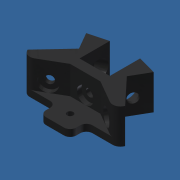
# Autodesk Inventor part: hexagon_top_v_2_0_x1
Saved by Autodesk Inventor 2014 SP2 (Build 180246200, 246)
## iProperties
Created: 2013-09-01
Part Number: hexagon_top_v_2_0_x1
Material: ABS-Kunststoff - Schwarz
Document SubType Name: Modeling
Designer: gerdkeller
Density: 1.06 g/cm^3
Appearance: Glatt - weiß(2)
Author: gerdkeller
Autodesk Inventor part; units mm, degrees
sketch "Skizze1" plane through (0, 0, 0) normal (0, 0, 1) x (1, 0, 0)
  line L0 (10, 10) -> (10, -10)
  line L1 (10, -10) -> (-10, -10)
  line L2 (-10, -10) -> (-10, 10)
  line L3 (0, 8) -> (17.3205, -2) construction
  line L4 (0, 8) -> (20, 8) construction
  line L5 (17.3205, -2) -> (12.3205, -10.6603) construction
  line L6 (17.3205, -2) -> (22.3205, 6.6603) construction
  line L7 (22.3205, 6.6603) -> (12.3205, -10.6603)
  line L8 (12.3205, -10.6603) -> (32.2391, -22.1603)
  line L9 (10, -10) -> (10, -20) construction
  line L10 (-10, -10) -> (-10, -20) construction
  line L11 (29.2391, -27.3564) -> (10, -16.2487)
  line L12 (10, -16.2487) -> (-10, -16.2487)
  line L13 (29.2391, -27.3564) -> (32.2391, -22.1603)
  line L14 (10, 10) -> (22.3205, 6.6603)
  line L15 (0, 17.4713) -> (0, -34.8277) projected
  line L16 (-45.1347, 0) -> (45.1347, 0) projected
  line L17 (-17.3205, -2) -> (-12.3205, -10.6603) construction
  line L18 (-17.3205, -2) -> (-22.3205, 6.6603) construction
  line L19 (-22.3205, 6.6603) -> (-12.3205, -10.6603)
  line L20 (-12.3205, -10.6603) -> (-32.2391, -22.1603)
  line L21 (-29.2391, -27.3564) -> (-10, -16.2487)
  line L22 (-29.2391, -27.3564) -> (-32.2391, -22.1603)
  line L23 (-10, 10) -> (-22.3205, 6.6603)
  point P0 (0, 0)
  dimension "d0" = 20
  dimension "d2" = 20
  dimension "d3" = 30
  dimension "d4" = 10
  dimension "d5" = 10
  dimension "d6" = 23
  dimension "d7" = 6
  dimension "d28" = 10
  dimension "d29" = 8
  dimension "d30" = 16.2487
  dimension "d31" = 30
  dimension "d32" = 14.833
  dimension "d101" = 17.3205
  constraints: 44 end point, 5 symmetric about line, 3 parallel, 3 perpendicular, 2 collinear, 2 point on line, 1 equal length, 1 horizontal, 2 other
  measures "d0" distance between parallel lines of L0 L2
  measures "d2" distance of L3.start L3.end
  measures "d3" angle of L3 L4
  measures "d4" distance of L3.end L5.end
  measures "d5" distance of L3.end L6.end
  measures "d6" distance of L5.end L8.end
  measures "d7" distance between parallel lines of L8 L11
  measures "d28" distance between parallel lines of L1 L16
  measures "d29" distance from line of L16 L3.start
  measures "d30" distance between parallel lines of L12 L16
  measures "d31" angle of L16 L8
  measures "d32" angle of L3 L14
  measures "d101" distance from line of L3.end L15
extrude "Extrusion1" add sketch "Skizze1" along normal blind 40 contours L14 L7 L16 L0 | L16 L7 L8 L13 L11 L12 L15 L1 L0 | L15 L12 L21 L22 L20 L19 L16 L2 L1 | L16 L19 L23 L2
sketch "Skizze5" plane through (0, 0, 0) normal (0, 0, -1) x (-1, 0, 0)
  line L0 (10, 10) -> (10, -10) projected
  line L1 (10, -10) -> (-10, -10) projected
  line L2 (-10, -10) -> (-10, 10) projected
  line L3 (-10, 10) -> (-22.3205, 6.6603) projected
  line L4 (-22.3205, 6.6603) -> (-12.3205, -10.6603) projected
  line L5 (-12.3205, -10.6603) -> (-32.2391, -22.1603) projected
  line L6 (-32.2391, -22.1603) -> (-29.2391, -27.3564) projected
  line L7 (-29.2391, -27.3564) -> (-10, -16.2487) projected
  line L8 (-10, -16.2487) -> (10, -16.2487) projected
  line L9 (10, -16.2487) -> (29.2391, -27.3564) projected
  line L10 (29.2391, -27.3564) -> (32.2391, -22.1603) projected
  line L11 (32.2391, -22.1603) -> (12.3205, -10.6603) projected
  line L12 (12.3205, -10.6603) -> (22.3205, 6.6603) projected
  line L13 (22.3205, 6.6603) -> (10, 10) projected
  line L14 (-10, 10) -> (10, 10)
  line L15 (32.2391, -22.1603) -> (42.2391, -4.8397)
  line L16 (42.2391, -4.8397) -> (22.3205, 6.6603)
  line L17 (-32.2391, -22.1603) -> (-42.2391, -4.8397)
  line L18 (-42.2391, -4.8397) -> (-22.3205, 6.6603)
  point P0 (0, 0)
  dimension "d33" = 20
  dimension "d34" = 20
  constraints: 10 end point, 2 parallel, 1 perpendicular
  measures "d33" distance of L10.end L15.end
  measures "d34" distance of L5.end L17.end
extrude "Extrusion5" add sketch "Skizze5" along normal blind 6
sketch "Skizze6" plane through (0, 0, 0) normal (0, 0, 1) x (1, 0, 0)
  line L0 (42.2391, -4.8397) -> (32.2391, -22.1603) projected
  line L1 (22.3205, 6.6603) -> (42.2391, -4.8397) projected
  circle A0 centre (27.2798, -7.75) radius 2.6
  point P0 (0, 0)
  dimension "d37" = 5.2
  dimension "d38" = 10
  dimension "d39" = 11.5
  constraints: 1 centre point
  measures "d37" diameter of A0
  measures "d38" distance from line of A0.centre L1
  measures "d39" distance from line of L0 A0.centre
extrude "Extrusion6" cut sketch "Skizze6" against normal blind 6
sketch "Skizze7" plane through (0, 0, -6) normal (0, 0, -1) x (-1, 0, 0)
  circle A0 centre (-27.2798, -7.75) radius 2.6 projected
  circle A1 centre (-27.2798, -7.75) radius 5.5
  point P0 (0, 0)
  dimension "d42" = 11
  constraints: 1 centre point, 1 coincident
  measures "d42" diameter of A1
extrude "Extrusion7" cut sketch "Skizze7" against normal blind 3
sketch "Skizze8" plane through (27.2798, -7.75, -3) normal (0, 0, -1) x (-1, 0, 0)
  circle A0 centre (0, 0) radius 2.6 projected
  point P0 (27.2798, 7.75)
extrude "Extrusion8" add sketch "Skizze8" against normal blind 0.4
mirror "Spiegeln1" about plane through (0, 0, 0) normal (1, 0, 0) of "Extrusion6", "Extrusion7", "Extrusion8"
sketch "Skizze9" plane through (12.3205, -10.6603, 40) normal (0.5, 0.8660254, 0) x (0.8660254, -0.5, 0)
  circle A0 centre (11.5, 10) radius 2.6
  point P0 (-16, 40)
  dimension "d47" = 5.2
  constraints: 1 centre point
  measures "d47" diameter of A0
extrude "Extrusion9" cut sketch "Skizze9" against normal blind 6
sketch "Skizze10" plane through (29.2391, -27.3564, -6) normal (-0.5, -0.8660254, 0) x (0.8660254, -0.5, 0)
  circle A0 centre (-11.5, 36) radius 2.6 projected
  circle A1 centre (-11.5, 36) radius 5.5
  point P0 (-39, 6)
  dimension "d50" = 11
  constraints: 1 centre point, 1 coincident
  measures "d50" diameter of A1
extrude "Extrusion10" cut sketch "Skizze10" against normal blind 3
mirror "Spiegeln2" about plane through (0, 0, 0) normal (1, 0, 0) of "Extrusion10", "Extrusion9"
sketch "Skizze12" plane through (0, 0, -6) normal (0, 0, -1) x (-1, 0, 0)
  line L0 (-10, -16.2487) -> (10, -16.2487) projected
  line L1 (10, 10) -> (-10, 10) projected
  line L2 (-10, -16.2487) -> (-10, -36.2487)
  line L3 (-10, -36.2487) -> (10, -36.2487)
  line L4 (10, -36.2487) -> (10, -16.2487)
  point P0 (0, 0)
  dimension "d55" = 20
  constraints: 6 end point, 3 perpendicular
  measures "d55" distance of L0.start L2.end
extrude "Extrusion12" add sketch "Skizze12" against normal blind 6
sketch "Skizze13" plane through (0, 0, 0) normal (0, 0, 1) x (1, 0, 0)
  line L0 (-10, -36.2487) -> (10, -36.2487) projected
  circle A0 centre (0, -26.2487) radius 2.6
  point P0 (0, 0)
  dimension "d58" = 5.2
  dimension "d59" = 10
  constraints: 1 centre point
  measures "d58" diameter of A0
  measures "d59" distance from line of L0 A0.centre
extrude "Extrusion13" cut sketch "Skizze13" against normal blind 6
sketch "Skizze14" plane through (0, 0, -6) normal (0, 0, -1) x (-1, 0, 0)
  circle A0 centre (0, -26.2487) radius 2.6 projected
  circle A1 centre (0, -26.2487) radius 5.5
  point P0 (0, 0)
  dimension "d62" = 11
  constraints: 1 centre point, 1 coincident
  measures "d62" diameter of A1
extrude "Extrusion14" cut sketch "Skizze14" against normal blind 3
sketch "Skizze15" plane through (0, -26.2487, -3) normal (0, 0, -1) x (-1, 0, 0)
  circle A0 centre (0, 0) radius 2.6 projected
  point P0 (0, 26.2487)
extrude "Extrusion15" add sketch "Skizze15" against normal blind 0.4
fillet "Rundung1" radius 5 2 edges at (10, -16.2487, -3) (-10, -16.2487, -3)
sketch "Skizze16" plane through (0, 0, 0) normal (0, 0, 1) x (1, 0, 0)
  circle A0 centre (0, 0) radius 2.6
  dimension "d68" = 5.2
  constraints: 1 centre point, 1 coincident
  measures "d68" diameter of A0
extrude "Extrusion16" cut sketch "Skizze16" against normal blind 6
sketch "Skizze17" plane through (0, 0, -6) normal (0, 0, -1) x (-1, 0, 0)
  circle A0 centre (0, 0) radius 2.6 projected
  circle A1 centre (0, 0) radius 5.5
  dimension "d71" = 11
  constraints: 1 centre point, 1 coincident
  measures "d71" diameter of A1
extrude "Extrusion17" cut sketch "Skizze17" against normal blind 3
sketch "Skizze18" plane through (0, 0, -3) normal (0, 0, -1) x (-1, 0, 0)
  circle A0 centre (0, 0) radius 2.6 projected
extrude "Extrusion18" add sketch "Skizze18" against normal blind 0.4
sketch "Skizze19" plane through (-10, -16.2487, 40) normal (0, -1, 0) x (1, 0, 0)
  circle A0 centre (10, -10) radius 2.6
  point P0 (10, -40)
  dimension "d76" = 5.2
  constraints: 1 centre point
  measures "d76" diameter of A0
extrude "Extrusion19" cut sketch "Skizze19" against normal blind 7
sketch "Skizze20" plane through (-10, -16.2487, 40) normal (0, -1, 0) x (1, 0, 0)
  circle A0 centre (10, -10) radius 2.6 projected
  circle A1 centre (10, -10) radius 5.5
  point P0 (10, -40)
  dimension "d79" = 11
  constraints: 1 centre point, 1 coincident
  measures "d79" diameter of A1
extrude "Extrusion20" cut sketch "Skizze20" against normal blind 3
sketch "Skizze21" plane through (-10, -16.2487, 40) normal (0, -1, 0) x (1, 0, 0)
  circle A0 centre (10, -10) radius 5.5 projected
  circle A1 centre (10, -30) radius 2.6
  point P0 (10, -40)
  dimension "d82" = 5.2
  dimension "d83" = 20
  constraints: 1 centre point
  measures "d82" diameter of A1
  measures "d83" distance of A1.centre A0.centre
extrude "Extrusion21" cut sketch "Skizze21" against normal blind 10 contours A1
sketch "Skizze22" plane through (-10, -16.2487, 40) normal (0, -1, 0) x (1, 0, 0)
  circle A0 centre (10, -30) radius 2.6 projected
  circle A1 centre (10, -30) radius 5.5
  point P0 (10, -40)
  dimension "d86" = 11
  constraints: 1 centre point, 1 coincident
  measures "d86" diameter of A1
extrude "Extrusion22" cut sketch "Skizze22" against normal blind 3
sketch "Skizze23" plane through (29.2391, -27.3564, -6) normal (-0.5, -0.8660254, 0) x (0.8660254, -0.5, 0)
  line L0 (0, 46) -> (0, 0) projected
  circle A0 centre (-11.5, 36) radius 5.5 projected
  circle A1 centre (-11.5, 16) radius 2.6
  point P0 (-39, 6)
  dimension "d89" = 5.2
  dimension "d90" = 20
  dimension "d91" = 11.5
  constraints: 1 centre point
  measures "d89" diameter of A1
  measures "d90" distance of A1.centre A0.centre
  measures "d91" distance from line of L0 A1.centre
extrude "Extrusion23" cut sketch "Skizze23" against normal blind 10 contours A1
sketch "Skizze24" plane through (29.2391, -27.3564, -6) normal (-0.5, -0.8660254, 0) x (0.8660254, -0.5, 0)
  circle A0 centre (-11.5, 16) radius 2.6 projected
  circle A1 centre (-11.5, 16) radius 5.5
  point P0 (-39, 6)
  dimension "d94" = 11
  constraints: 1 centre point, 1 coincident
  measures "d94" diameter of A1
extrude "Extrusion24" cut sketch "Skizze24" against normal blind 3
mirror "Spiegeln3" about plane through (0, 0, 0) normal (1, 0, 0) of "Extrusion24", "Extrusion23"
fillet "Rundung2" radius 5 6 edges at (-29.2391, -27.3564, 17) (29.2391, -27.3564, 17) (10, -36.2487, -3) (-10, -36.2487, -3) (42.2391, -4.8397, -3) (-42.2391, -4.8397, -3)
sketch "Skizze25" plane through (0, 0, 40) normal (0, 0, 1) x (1, 0, 0)
  arc A0 (24.909, -24.8564) -> (31.7391, -23.0263) centre (27.409, -20.5263) ccw projected
  line L0 (31.7391, -23.0263) -> (32.2391, -22.1603) projected
  line L1 (32.2391, -22.1603) -> (12.3205, -10.6603) projected
  line L2 (12.3205, -10.6603) -> (22.3205, 6.6603) projected
  line L3 (22.3205, 6.6603) -> (10, 10) projected
  line L4 (10, 10) -> (10, -10) projected
  line L5 (10, -10) -> (-10, -10) projected
  line L6 (-10, -10) -> (-10, 10) projected
  line L7 (-10, 10) -> (-22.3205, 6.6603) projected
  line L8 (-22.3205, 6.6603) -> (-12.3205, -10.6603) projected
  line L9 (-12.3205, -10.6603) -> (-32.2391, -22.1603) projected
  line L10 (-32.2391, -22.1603) -> (-31.7391, -23.0263) projected
  arc A1 (-31.7391, -23.0263) -> (-24.909, -24.8564) centre (-27.409, -20.5263) ccw projected
  line L11 (-24.909, -24.8564) -> (-10, -16.2487) projected
  line L12 (-10, -16.2487) -> (10, -16.2487) projected
  line L13 (10, -16.2487) -> (24.909, -24.8564) projected
  point P0 (0, 0)
extrude "Extrusion25" cut sketch "Skizze25" against normal blind 20
ref_plane "Arbeitsebene1" through (0, 0, 0) normal (0, 0, 1) x (1, 0, 0)
split "Trennen1" plane through (0, 0, 0) removes the side toward (0, 0, -1)
sketch "Skizze26" plane through (-22.3205, 6.6603, 0) normal (-0.8660254, -0.5, 0) x (0, 0, 1)
  line L0 (0, 0) -> (20, -20) construction
  point P0 (0, -16.9282)
  point P1 (10, -10)
  constraints: 2 end point, 1 midpoint
hole "Bohrung1" at (-17.3205, -2, 10) direction (0.8660254, 0.5, 0) diameter 6.4 end through all
ref_plane "Arbeitsebene2" through (-10, 10, 0) normal (-0.8660254, -0.5, 0) x (0, 0, 1)
sketch "Skizze27" plane through (-10, 10, 0) normal (-0.8660254, -0.5, 0) x (0, 0, 1)
  circle A0 centre (10, -6.7321) radius 3.2 projected
  point P0 (0, -13.6603)
ref_plane "Arbeitsebene3" through (0, -10, 10) normal (0, 0, -1) x (0, -1, 0)
sketch "Skizze28" plane through (0, -10, 10) normal (0, 0, -1) x (0, -1, 0)
  line L0 (-20, 10) -> (-16.6603, 22.3205) projected
  line L1 (-16.6603, 22.3205) -> (-10.7713, 18.9205) projected
  line L2 (-10.7713, 18.9205) -> (-15.9215, 10) projected
  line L3 (-15.9215, 10) -> (-20, 10) projected
  line L4 (12.1603, 32.2391) -> (13.0263, 31.7391) projected
  arc A0 (14.8564, 24.909) -> (13.0263, 31.7391) centre (10.5263, 27.409) ccw projected
  line L5 (14.8564, 24.909) -> (14.3564, 24.0429) projected
  line L6 (14.3564, 24.0429) -> (11.7583, 25.5429) projected
  line L7 (11.7583, 25.5429) -> (10.3083, 23.0315) projected
  line L8 (10.3083, 23.0315) -> (7.7103, 24.5315) projected
  line L9 (7.7103, 24.5315) -> (12.1603, 32.2391) projected
  line L10 (11.7583, -25.5429) -> (14.3564, -24.0429) projected
  line L11 (14.3564, -24.0429) -> (14.8564, -24.909) projected
  arc A1 (13.0263, -31.7391) -> (14.8564, -24.909) centre (10.5263, -27.409) ccw projected
  line L12 (13.0263, -31.7391) -> (12.1603, -32.2391) projected
  line L13 (12.1603, -32.2391) -> (7.7103, -24.5315) projected
  line L14 (7.7103, -24.5315) -> (10.3083, -23.0315) projected
  line L15 (10.3083, -23.0315) -> (11.7583, -25.5429) projected
  line L16 (6.2487, 5.5) -> (3.2487, 5.5) projected
  line L17 (3.2487, 5.5) -> (3.2487, 2.6) projected
  line L18 (3.2487, 2.6) -> (0, 2.6) projected
  line L19 (0, 2.6) -> (0, 10) projected
  line L20 (0, 10) -> (-8.5315, 10) projected
  line L21 (-8.5315, 10) -> (-5.2287, 15.7205) projected
  line L22 (-5.2287, 15.7205) -> (0.6603, 12.3205) projected
  line L23 (0.6603, 12.3205) -> (5.1103, 20.0281) projected
  line L24 (5.1103, 20.0281) -> (7.7083, 18.5281) projected
  line L25 (7.7083, 18.5281) -> (6.2583, 16.0167) projected
  line L26 (6.2583, 16.0167) -> (8.8564, 14.5167) projected
  line L27 (8.8564, 14.5167) -> (6.2487, 10) projected
  line L28 (6.2487, 10) -> (6.2487, 5.5) projected
  line L29 (3.2487, -5.5) -> (6.2487, -5.5) projected
  line L30 (6.2487, -5.5) -> (6.2487, -10) projected
  line L31 (6.2487, -10) -> (8.8564, -14.5167) projected
  line L32 (8.8564, -14.5167) -> (6.2583, -16.0167) projected
  line L33 (6.2583, -16.0167) -> (7.7083, -18.5281) projected
  line L34 (7.7083, -18.5281) -> (5.1103, -20.0281) projected
  line L35 (5.1103, -20.0281) -> (0.6603, -12.3205) projected
  line L36 (0.6603, -12.3205) -> (-16.6603, -22.3205) projected
  line L37 (-16.6603, -22.3205) -> (-20, -10) projected
  line L38 (-20, -10) -> (0, -10) projected
  line L39 (0, -10) -> (0, -2.6) projected
  line L40 (0, -2.6) -> (3.2487, -2.6) projected
  line L41 (3.2487, -2.6) -> (3.2487, -5.5) projected
  line L42 (-39.8575, -37.8582) -> (11.9252, 51.832) projected
  line L43 (-7.455, 18.2645) -> (-15.7195, 16.05)
  line L44 (-15.7195, 16.05) -> (-19.2124, 10)
  line L45 (-19.2124, 10) -> (-8.7335, 3.95)
  line L46 (-8.7335, 3.95) -> (-5.2406, 10)
  line L47 (-5.2406, 10) -> (-7.455, 18.2645)
  line L48 (-15.7195, 16.05) -> (-5.2406, 10)
  line L49 (-7.455, 18.2645) -> (-13.973, 6.975)
  point P0 (-10, 0)
  dimension "d110" = 12.1
  constraints: 15 end point, 3 perpendicular, 3 point on line, 1 midpoint, 1 parallel, 2 other
  measures "d110" distance between parallel lines of L44 L46
revolve "Umdrehung1" cut sketch "Skizze28" angle 360 about axis through (48.7451, 36.143, 10) along (-0.8660254, -0.5, 0) contours L44 L48 L2 L3 | L3 L2 L48 L42 L45 | L43 L2 L48 | L43 L42 L48 L2
ref_plane "Arbeitsebene4" through (0, -10, 10) normal (1, 0, 0) x (0, -1, 0)
mirror "Spiegeln4" about plane through (0, -10, 10) normal (1, 0, 0) of "Umdrehung1", "Bohrung1"
sketch "Skizze32" plane through (10, -10, 0) normal (0, 0, -1) x (-1, 0, 0)
  arc A0 (34.909, -14.8564) -> (41.7391, -13.0263) centre (37.409, -10.5263) ccw projected
  arc A1 (-21.7391, -13.0263) -> (-14.909, -14.8564) centre (-17.409, -10.5263) ccw projected
  line L0 (0, -6.2487) -> (-14.909, -14.8564) projected
  line L1 (20, -6.2487) -> (0, -6.2487) projected
  line L2 (34.909, -14.8564) -> (20, -6.2487) projected
  line L3 (-17.409, -15.5263) -> (37.409, -15.5263)
  point P0 (10, 10)
  constraints: 2 end point, 2 point on circle, 1 parallel, 1 tangent
extrude "Extrusion28" add sketch "Skizze32" against normal blind 4.5
sketch "Skizze33" plane through (0, 0, 20) normal (0, 0, 1) x (1, 0, 0)
  arc A0 (24.909, -24.8564) -> (31.7391, -23.0263) centre (27.409, -20.5263) ccw projected
  line L0 (32.2391, -22.1603) -> (31.7391, -23.0263) projected
  line L1 (12.3205, -10.6603) -> (32.2391, -22.1603) projected
  line L2 (22.3205, 6.6603) -> (12.3205, -10.6603) projected
  line L3 (10, 10) -> (22.3205, 6.6603) projected
  line L4 (10, -10) -> (10, 10) projected
  line L5 (-10, -10) -> (10, -10) projected
  line L6 (-10, 10) -> (-10, -10) projected
  line L7 (-22.3205, 6.6603) -> (-10, 10) projected
  line L8 (-12.3205, -10.6603) -> (-22.3205, 6.6603) projected
  line L9 (-32.2391, -22.1603) -> (-12.3205, -10.6603) projected
  line L10 (-31.7391, -23.0263) -> (-32.2391, -22.1603) projected
  arc A1 (-31.7391, -23.0263) -> (-24.909, -24.8564) centre (-27.409, -20.5263) ccw projected
  line L11 (-10, -16.2487) -> (-24.909, -24.8564) projected
  line L12 (10, -16.2487) -> (-10, -16.2487) projected
  line L13 (24.909, -24.8564) -> (10, -16.2487) projected
  line L14 (-32.2391, -22.1603) -> (-15.8205, -4.5981)
  line L15 (32.2391, -22.1603) -> (15.8205, -4.5981)
  point P0 (0, 0)
  dimension "d121" = 7
  dimension "d122" = 7
  constraints: 4 end point, 2 point on line
  measures "d121" distance from line of L14.end L9
  measures "d122" distance from line of L15.end L1
extrude "Extrusion29" add sketch "Skizze33" along normal blind 3
sketch "Skizze34" plane through (10, -10, 4.5) normal (0, 0, 1) x (1, 0, 0)
  line L0 (-20, -6.2487) -> (-10, -6.2487) projected
  line L1 (-20, -6.2487) -> (0, -6.2487)
  line L2 (0, -6.2487) -> (0, -26.2487)
  line L3 (0, -26.2487) -> (-20, -26.2487)
  line L4 (-20, -26.2487) -> (-20, -6.2487)
  point P0 (-10, 10)
  dimension "d125" = 20
  constraints: 8 end point, 2 parallel, 1 horizontal, 1 perpendicular
  measures "d125" distance between parallel lines of L3 L0
extrude "Extrusion30" add sketch "Skizze34" against normal up to surface (4.5 mm away)
sketch "Skizze35" plane through (10, -10, 4.5) normal (0, 0, 1) x (1, 0, 0)
  line L0 (0, -6.2487) -> (-20, -26.2487)
  point P0 (-10, 10)
  point P1 (-10, -16.2487)
  constraints: 2 end point, 1 midpoint
hole "Bohrung2" at (0, -26.2487, 4.5) direction (0, 0, -1) diameter 4 end through all
fillet "Rundung4" radius 4 4 edges at (-10, -25.5263, 2.25) (-10, -36.2487, 2.25) (10, -36.2487, 2.25) (10, -25.5263, 2.25)
equation "\"d122\" = d121"
